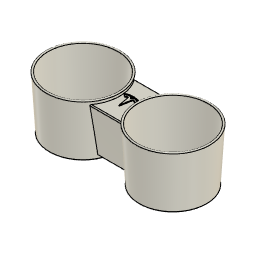
CupHolders (Autodesk Fusion 360 design; units mm, degrees)
Autodesk Fusion 360 part; units mm, degrees
note: some values were not read from the file. Set by a fixed rule: which face or edge a step refers to.
sketch "Bottom" plane through (0, 0, 0) normal (0, 0, 1) x (1, 0, 0)
  circle A0 centre (50, 0) radius 37.5
  line L0 (0, 0) -> (50, 0) construction
  line L1 (0, 2.5) -> (0, 20)
  dimension "d5" = 75
  dimension "d50" = 50
  constraint coincident L0.start origin
  constraint horizontal L0
  constraint coincident A0.centre L0.end
  measures "d5" diameter of A0
  measures "d50" distance of L0.start A0.centre
sketch "Base Ring" plane through (0, 0, 0) normal (0, 0, 1) x (1, 0, 0)
  line L0 (78.4489, -12.3251) -> (78.8316, -11.4012)
  line L1 (61.4012, 28.8316) -> (62.5493, 31.6032)
  line L2 (50.5, -31) -> (50.5, -34)
  line L3 (78.8316, -11.4012) -> (81.6032, -12.5493)
  line L4 (18.3968, -12.5493) -> (21.1684, -11.4012)
  line L5 (81, -0.5) -> (81, 0.5)
  line L6 (37.4507, 31.6032) -> (38.5988, 28.8316)
  line L7 (61.4012, -28.8316) -> (62.3251, -28.4489)
  line L8 (27.7261, 21.5668) -> (25.6048, 23.6881)
  line L9 (71.5668, 22.2739) -> (73.6881, 24.3952)
  line L10 (36.5268, -31.2206) -> (37.6749, -28.4489)
  line L11 (73.6881, 24.3952) -> (74.3952, 23.6881)
  line L12 (49.5, -31) -> (50.5, -31)
  line L13 (36.5268, 31.2206) -> (37.4507, 31.6032)
  line L14 (37.4507, -31.6032) -> (36.5268, -31.2206)
  line L15 (50, 30) -> (50, 31) construction
  line L16 (50.5, 31) -> (49.5, 31)
  line L17 (49.5, 31) -> (49.5, 34)
  line L18 (18.3968, 12.5493) -> (18.7794, 13.4732)
  line L19 (25.6048, 23.6881) -> (26.3119, 24.3952)
  line L20 (21.5511, 12.3251) -> (21.1684, 11.4012)
  circle A0 centre (50, 0) radius 30
  line L21 (50.5, 34) -> (50.5, 31)
  line L22 (16, -0.5) -> (16, 0.5)
  line L23 (19, -0.5) -> (16, -0.5)
  line L24 (16, 0.5) -> (19, 0.5)
  line L25 (25.6048, -23.6881) -> (27.7261, -21.5668)
  line L26 (18.7794, 13.4732) -> (21.5511, 12.3251)
  line L27 (49.5, 34) -> (50.5, 34)
  line L28 (63.4732, 31.2206) -> (62.3251, 28.4489)
  line L29 (28.4332, -22.2739) -> (26.3119, -24.3952)
  line L30 (62.5493, 31.6032) -> (63.4732, 31.2206)
  line L31 (21.1684, -11.4012) -> (21.5511, -12.3251)
  line L32 (26.3119, -24.3952) -> (25.6048, -23.6881)
  line L33 (28.4332, 22.2739) -> (27.7261, 21.5668)
  line L34 (19, 0.5) -> (19, -0.5)
  line L35 (21.1684, 11.4012) -> (18.3968, 12.5493)
  line L36 (27.7261, -21.5668) -> (28.4332, -22.2739)
  line L37 (71.5668, -22.2739) -> (72.2739, -21.5668)
  line L38 (63.4732, -31.2206) -> (62.5493, -31.6032)
  line L39 (74.3952, -23.6881) -> (73.6881, -24.3952)
  line L40 (78.4489, 12.3251) -> (81.2206, 13.4732)
  line L41 (73.6881, -24.3952) -> (71.5668, -22.2739)
  line L42 (78.8316, 11.4012) -> (78.4489, 12.3251)
  line L43 (81.6032, 12.5493) -> (78.8316, 11.4012)
  line L44 (72.2739, -21.5668) -> (74.3952, -23.6881)
  line L45 (62.3251, -28.4489) -> (63.4732, -31.2206)
  line L46 (81.2206, 13.4732) -> (81.6032, 12.5493)
  line L47 (72.2739, 21.5668) -> (71.5668, 22.2739)
  line L48 (49.5, -34) -> (49.5, -31)
  line L49 (26.3119, 24.3952) -> (28.4332, 22.2739)
  line L50 (37.6749, 28.4489) -> (36.5268, 31.2206)
  line L51 (38.5988, 28.8316) -> (37.6749, 28.4489)
  line L52 (62.3251, 28.4489) -> (61.4012, 28.8316)
  line L53 (18.7794, -13.4732) -> (18.3968, -12.5493)
  line L54 (37.6749, -28.4489) -> (38.5988, -28.8316)
  line L55 (84, 0.5) -> (84, -0.5)
  line L56 (38.5988, -28.8316) -> (37.4507, -31.6032)
  line L57 (50.5, -34) -> (49.5, -34)
  line L58 (74.3952, 23.6881) -> (72.2739, 21.5668)
  line L59 (81, 0.5) -> (84, 0.5)
  line L60 (81.6032, -12.5493) -> (81.2206, -13.4732)
  line L61 (84, -0.5) -> (81, -0.5)
  line L62 (62.5493, -31.6032) -> (61.4012, -28.8316)
  line L63 (21.5511, -12.3251) -> (18.7794, -13.4732)
  line L64 (81.2206, -13.4732) -> (78.4489, -12.3251)
  line L65 (0, 0) -> (50, 0) construction
  point P0 (50, 0)
  point P1 (28.0797, 21.9203)
  point P2 (38.1368, 28.6403)
  point P3 (50, 0)
  point P4 (21.3597, -11.8632)
  point P5 (28.0797, -21.9203)
  point P6 (38.1368, -28.6403)
  point P7 (81, 0)
  point P8 (78.6403, -11.8632)
  point P9 (19, 0)
  point P10 (21.3597, 11.8632)
  point P11 (78.6403, 11.8632)
  point P12 (71.9203, 21.9203)
  point P13 (61.8632, 28.6403)
  point P14 (50, -31)
  point P15 (61.8632, -28.6403)
  point P16 (71.9203, -21.9203)
  dimension "d44" = 360
  dimension "d45" = 1
  dimension "d46" = 3
  dimension "d47" = 1
  dimension "d48" = 50
  dimension "d49" = 60
  constraint coincident P3 P0
  constraint coincident L15.start A0
  constraint vertical L15
  constraint coincident P3 L15
  constraint horizontal L27
  constraint vertical L21
  constraint horizontal L16
  constraint vertical L17
  constraint midpoint L15.end L16
  constraint coincident L65.start origin
  constraint horizontal L65
  measures "d45" distance of L15.end L15.start
  measures "d46" distance of L16.start L21.start
  measures "d47" distance of L17.end L21.start
  measures "d48" distance of L65.start P3
  measures "d49" diameter of A0
sketch "Base Logo" plane through (0, 0, 0) normal (0, 0, 1) x (1, 0, 0)
  line L0 (48.0037, -22.4312) -> (53.2176, 6.8922)
  spline S0 degree 3 poles (53.2176, 6.8922) (58.1874, 6.8922) (59.755, 6.3472) (59.9813, 4.1228) knots 0 0 0 0 1 1 1 1
  spline S1 degree 2 poles (59.9813, 4.1228) (63.3152, 5.3659) (64.9967, 7.8905) knots 0 0 0 1 1 1
  spline S2 degree 2 poles (64.9967, 7.8905) (58.435, 10.9311) (51.8421, 11.0682) knots 0 0 0 1 1 1
  line L1 (51.8421, 11.0682) -> (47.995, 6.3825)
  line L2 (47.995, 6.3825) -> (48.0037, 6.3831)
  line L3 (48.0037, 6.3831) -> (44.1566, 11.0689)
  spline S3 degree 2 poles (44.1566, 11.0689) (37.5635, 10.9317) (31.0027, 7.8911) knots 0 0 0 1 1 1
  spline S4 degree 2 poles (31.0027, 7.8911) (32.6827, 5.3665) (36.0179, 4.1234) knots 0 0 0 1 1 1
  spline S5 degree 3 poles (36.0179, 4.1234) (36.2456, 6.3479) (37.8113, 6.8929) (42.7477, 6.8964) knots 0 0 0 0 1 1 1 1
  line L4 (42.7477, 6.8964) -> (48.0037, -22.4312)
  spline S6 degree 3 poles (48.0016, 12.4216) (53.3058, 12.4622) (59.377, 11.6011) (65.5921, 8.8923) knots 0 0 0 0 1 1 1 1
  spline S7 degree 2 poles (65.5921, 8.8923) (66.4227, 10.3874) (66.6363, 11.0482) knots 0 0 0 1 1 1
  spline S8 degree 3 poles (66.6363, 11.0482) (59.8423, 13.7361) (53.4798, 14.656) (48.0009, 14.6791) knots 0 0 0 0 1 1 1 1
  spline S9 degree 3 poles (48.0009, 14.6791) (42.5223, 14.656) (36.16, 13.736) (29.3669, 11.0482) knots 0 0 0 0 1 1 1 1
  spline S10 degree 2 poles (29.3669, 11.0482) (29.67, 10.2343) (30.4104, 8.8923) knots 0 0 0 1 1 1
  spline S11 degree 3 poles (30.4104, 8.8923) (36.6243, 11.6011) (42.6966, 12.4622) (48.0009, 12.4216) knots 0 0 0 0 1 1 1 1
  line L5 (48.0009, 12.4216) -> (48.0016, 12.4216)
sketch "Bridge" plane through (0, 0, 0) normal (1, 0, 0) x (0, 1, 0)
  line L0 (-16.5, 0) -> (16.5, 0) construction
  line L1 (0, 0) -> (0, 60) construction
  line L2 (-25.5, 60) -> (25.5, 60) construction
  line L3 (16.5, 0) -> (25.5, 60) construction
  line L4 (-16.5, 0) -> (-25.5, 60) construction
  line L5 (0, 0) -> (0, 4) construction
  line L6 (17.1, 4) -> (-17.1, 4)
  line L7 (0, 60) -> (0, 56) construction
  line L8 (24.9, 56) -> (-24.9, 56)
  line L9 (-24.9, 56) -> (-17.1, 4)
  line L10 (17.1, 4) -> (24.9, 56)
  dimension "d20" = 33
  dimension "d22" = 51
  dimension "d27" = 60
  dimension "d32" = 4
  dimension "d33" = 4
  constraint horizontal L0
  constraint vertical L1
  constraint horizontal L2
  constraint midpoint L1.end L2
  constraint midpoint L0 L1.start
  constraint coincident L1.start L5.start
  constraint vertical L5
  constraint coincident L3 L6.start
  constraint coincident L4 L6.end
  constraint parallel L0 L6
  constraint midpoint L5.end L6
  constraint vertical L7
  constraint coincident L3 L8.start
  constraint coincident L4 L8.end
  constraint midpoint L7.end L8
  measures "d20" distance of L0.start L0.end
  measures "d22" distance of L2.start L2.end
  measures "d27" distance of L1.start L1.end
  measures "d32" distance of L1.start L5.end
  measures "d33" distance of L1.end L7.end
sketch "Bridge Logo" plane through (0, 0, 0) normal (0, 0, 1) x (1, 0, 0)
  line L0 (-0.0062, -10.0802) -> (2.2946, 2.8596)
  spline S0 degree 3 poles (2.2946, 2.8596) (4.4877, 2.8596) (5.1795, 2.6191) (5.2793, 1.6376) knots 0 0 0 0 1 1 1 1
  spline S1 degree 2 poles (5.2793, 1.6376) (6.7505, 2.1861) (7.4925, 3.3002) knots 0 0 0 1 1 1
  spline S2 degree 2 poles (7.4925, 3.3002) (4.597, 4.6419) (1.6877, 4.7024) knots 0 0 0 1 1 1
  line L1 (1.6877, 4.7024) -> (-0.01, 2.6347)
  line L2 (-0.01, 2.6347) -> (-0.0062, 2.635)
  line L3 (-0.0062, 2.635) -> (-1.7038, 4.7027)
  spline S3 degree 2 poles (-1.7038, 4.7027) (-4.6132, 4.6422) (-7.5083, 3.3004) knots 0 0 0 1 1 1
  spline S4 degree 2 poles (-7.5083, 3.3004) (-6.767, 2.1864) (-5.2952, 1.6378) knots 0 0 0 1 1 1
  spline S5 degree 3 poles (-5.2952, 1.6378) (-5.1948, 2.6195) (-4.5039, 2.8599) (-2.3255, 2.8615) knots 0 0 0 0 1 1 1 1
  line L4 (-2.3255, 2.8615) -> (-0.0062, -10.0802)
  spline S6 degree 3 poles (-0.0071, 5.2997) (2.3336, 5.3176) (5.0127, 4.9376) (7.7553, 3.7422) knots 0 0 0 0 1 1 1 1
  spline S7 degree 2 poles (7.7553, 3.7422) (8.1218, 4.402) (8.2161, 4.6936) knots 0 0 0 1 1 1
  spline S8 degree 3 poles (8.2161, 4.6936) (5.218, 5.8797) (2.4103, 6.2857) (-0.0074, 6.2958) knots 0 0 0 0 1 1 1 1
  spline S9 degree 3 poles (-0.0074, 6.2958) (-2.425, 6.2857) (-5.2325, 5.8797) (-8.2302, 4.6936) knots 0 0 0 0 1 1 1 1
  spline S10 degree 2 poles (-8.2302, 4.6936) (-8.0965, 4.3344) (-7.7697, 3.7422) knots 0 0 0 1 1 1
  spline S11 degree 3 poles (-7.7697, 3.7422) (-5.0276, 4.9376) (-2.3481, 5.3176) (-0.0074, 5.2997) knots 0 0 0 0 1 1 1 1
  line L5 (-0.0074, 5.2997) -> (-0.0071, 5.2997)
ref_plane "WorkPlane1" through (0, 0, 60) normal (0, 0, 1) x (1, 0, 0)
sketch "Top" plane through (0, 0, 60) normal (0, 0, 1) x (1, 0, 0)
  line L0 (0, 0) -> (50, 0) construction
  circle A0 centre (50, 0) radius 41
  line L1 (0, 2.5) -> (0, 20)
  dimension "d11" = 50
  dimension "d12" = 82
  constraint coincident L0.start origin
  constraint horizontal L0
  constraint coincident L0.end A0.centre
  measures "d11" distance of L0.start L0.end
  measures "d12" diameter of A0
loft "Cup Loft" add profiles "Bottom", "Top" section 1 section 2 makes body 1
shell "Cup Shell" thickness 2 removed faces 1 at (60.805, 12.7422, 60) on bodies 1
extrude "Add Base Ring" add sketch "Base Ring" along normal blind 1 from surface at 2 bodies 1
extrude "Extrude3" cut sketch "Base Logo" against normal blind 1 from surface at 3 contours L1 L2 L3 | L0 S0 S1 S2 L1 L3 S3 S4 S5 L4 | S6 S7 S8 S9 S10 S11 bodies 1
mirror "Cup Mirror" about plane through (0, 0, 0) normal (1, 0, 0) of bodies 1 makes body 2
extrude "Extrude Bridge" add sketch "Bridge" along normal up to surface and the other way up to surface end surface at (70.2083, -35.0019, 50) second end surface at (-70.2083, -35.0019, 50) on bodies 1 2 bodies 1 2
extrude "Extrude4" add sketch "Bridge Logo" along normal blind 1 from surface at 56 contours L1 L2 L3 | L0 S0 S1 S2 L1 L3 S3 S4 S5 L4 | S6 S7 S8 S9 S10 S11 bodies 1
fillet "Fillet1" radius 1 10 edges at (13.6424, 14.1018, 60) (11.7746, 14.8262, 60) (0, -24.9, 56) (0, 24.9, 56) (-11.7746, 14.8262, 60) (-13.6424, 14.1018, 60) (15.0377, -13.5606, 0) (-15.0377, -13.5606, 0) (0, 17.1, 4) (0, -17.1, 4) on bodies 1 2
sketch "Profile Projection" plane through (0, 0, 0) normal (0, 0, 1) x (1, 0, 0)
  arc A0 (-17.3799, 24.7388) -> (-17.3799, -24.7388) centre (-50, 0) ccw
  line L0 (-17.3799, 24.7388) -> (17.3799, 24.7388)
  line L1 (-17.3799, -24.7388) -> (17.3799, -24.7388)
  arc A1 (90.94, 0) -> (17.3799, 24.7388) centre (50, 0) ccw
  arc A2 (17.3799, -24.7388) -> (90.94, 0) centre (50, 0) ccw
equation "CupBottomDiameter = 75 mm" comment "Diameter of exterior bottom of the cup"
equation "CupTopDiameter = 82 mm" comment "Diameter of exterior top of the cup"
equation "CupHeight = 60 mm" comment "Total exterior height of the cup holder"
equation "d5 = CupBottomDiameter"
equation "CupCenterFromMiddle = 50 mm" comment "Distance between middle of the bridge and center of either cup"
equation "CupWallThickness = 2 mm" comment "Thickness of cup walls (protruding inward)"
equation "d10 = CupHeight"
equation "d11 = CupCenterFromMiddle"
equation "d12 = CupTopDiameter"
equation "d14 = CupWallThickness"
equation "BridgeBottomWidth = 33 mm" comment "Width of bridge exterior at the very bottom of cup holder"
equation "BridgeTopWidth = 51 mm" comment "Width of bridge exterior at the very top of cup holder"
equation "d20 = BridgeBottomWidth"
equation "d22 = BridgeTopWidth"
equation "d27 = CupHeight"
equation "FiletDiameter = 1 mm" comment "Diameter of rounded corners wherever they are used"
equation "d30 = FiletDiameter"
equation "BridgeInset = 4 mm" comment "Air gaps above and below the bridge"
equation "d32 = BridgeInset"
equation "d33 = BridgeInset"
equation "BasePatternInset = 15 mm" comment "Distance between outer wall and where inner decorative ring begins"
equation "d48 = CupCenterFromMiddle"
equation "d49 = CupBottomDiameter - BasePatternInset"
equation "d50 = CupCenterFromMiddle"
equation "d52 = PatternThickness"
equation "PatternThickness = 1 mm" comment "Height of any patterns (e.g. logos)"
equation "d56 = -PatternThickness"
equation "d59 = PatternThickness"
named bodies: "Holders", "Left Cup"
